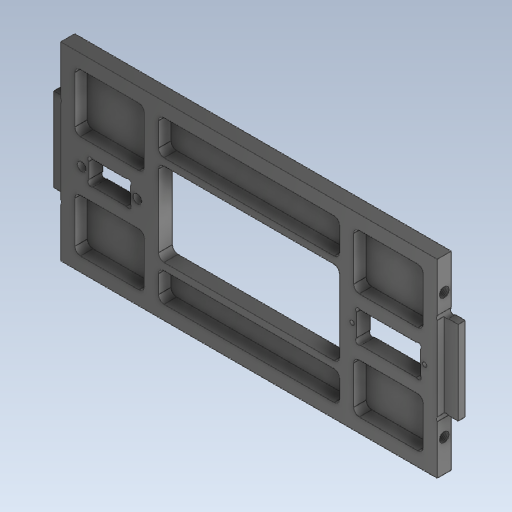
# Autodesk Inventor part: Cockpit_back_frame
Saved by Autodesk Inventor 2020 (Build 240168000, 168)
## iProperties
Part Number: Cockpit_back_frame
Material: アセタール樹脂、黒
Document SubType Name: Modeling
Designer: Masato Kubotera
Density: 1.425 g/cm^3
Appearance: 滑らか - 黒
Description: POM T5
Mass: 27.6157 g
Surface Area: 210.6 cm^2
Volume: 19.3794 cm^3
Author: Masato Kubotera
Autodesk Inventor part; units mm, degrees
ref_plane "XZ Plane" through (0, 0, 0) normal (0, 1, 0) x (-1, 0, 0)
ref_plane "XY Plane" through (0, 0, 0) normal (0, 0, 1) x (1, 0, 0)
derived "Cockpit_side_frame.ipt"
sketch "スケッチ2" plane through (0, 0, 0) normal (0, 1, 0) x (-1, 0, 0)
  line L0 (-23.5, -22.5) -> (-28.5, -27.5)
  line L1 (-28.5, -27.5) -> (-28.5, -91)
  line L2 (-28.5, -91) -> (-23.5, -96)
  line L3 (-23.5, -96) -> (35.75, -96)
  line L4 (37.75, -98) -> (37.75, -131)
  line L5 (37.75, -131) -> (42.75, -136)
  line L6 (42.75, -136) -> (83.5, -136)
  line L7 (88.5, -131) -> (88.5, -20)
  line L8 (88.5, -20) -> (86, -17.5)
  line L9 (86, -17.5) -> (80.25, -17.5)
  line L10 (80.25, -17.5) -> (80.25, -22.5)
  line L11 (80.25, -22.5) -> (73.9849, -22.5)
  line L12 (72.5, -21.0151) -> (72.5, -17.5)
  line L13 (72.5, -17.5) -> (64.5, -17.5)
  line L14 (64.5, -17.5) -> (64.5, -21.0151)
  line L15 (63.0151, -22.5) -> (-23.5, -22.5)
  line L16 (-25.25, -25) -> (-20.25, -25) construction
  line L17 (-20.25, -25) -> (-20.25, -93.5) construction
  line L18 (-20.25, -93.5) -> (-25.25, -93.5) construction
  line L19 (-25.25, -93.5) -> (-25.25, -25) construction
  line L20 (-26, -25) -> (-25.25, -25) construction
  line L21 (-25.25, -93.5) -> (-26, -93.5) construction
  line L22 (-26, -93.5) -> (-26, -25) construction
  line L23 (-20.25, -93.5) -> (80.25, -93.5) construction
  line L24 (-20.25, -88.5) -> (80.25, -88.5) construction
  line L25 (80.25, -22.5) -> (80.25, -90.5) construction
  line L26 (80.25, -90.5) -> (85.25, -90.5) construction
  line L27 (85.25, -90.5) -> (85.25, -22.5) construction
  line L28 (80.25, -88.5) -> (80.25, -93.5) construction
  line L29 (80.25, -91) -> (85.25, -91) construction
  line L30 (85.25, -91) -> (85.25, -133.5) construction
  line L31 (80.25, -91) -> (80.25, -133.5) construction
  line L32 (80.25, -133.5) -> (85.25, -133.5) construction
  line L33 (40.25, -133.5) -> (40.25, -128.5) construction
  line L34 (40.25, -128.5) -> (40.25, -93.5) construction
  line L35 (45.25, -93.5) -> (45.25, -128.5) construction
  line L36 (40.25, -128.5) -> (45.25, -128.5) construction
  line L37 (42.75, -128.5) -> (42.75, -93.5) construction
  line L38 (40.25, -128.5) -> (79.1145, -128.5) construction
  line L39 (79.1145, -128.5) -> (79.1145, -133.5) construction
  line L40 (79.1145, -133.5) -> (40.25, -133.5) construction
  line L41 (40.25, -131) -> (79.1145, -131) construction
  line L42 (82.75, -91) -> (82.75, -133.5) construction
  circle A0 centre (82.75, -131) radius 2
  arc A1 (80.25, -128.5) -> (85.25, -128.5) centre (82.75, -131) ccw construction
  line L43 (80.25, -91) -> (-20.25, -91) construction
  line L44 (42.75, -111) -> (45.25, -111) construction
  line L45 (59.6822, -128.5) -> (59.6822, -131) construction
  line L46 (42.7, -115.5651) -> (42.7, -106.4349)
  line L47 (45.3, -107.05) -> (45.3, -114.95)
  line L48 (45.3, -117.05) -> (42.7, -104.95) construction
  line L49 (42.7, -117.05) -> (45.3, -104.95) construction
  line L50 (55.7322, -128.45) -> (63.6322, -128.45)
  line L51 (64.2473, -131.05) -> (55.1172, -131.05)
  line L52 (53.6322, -128.45) -> (65.7322, -131.05) construction
  line L53 (65.7322, -128.45) -> (53.6322, -131.05) construction
  line L54 (42.75, -105) -> (45.25, -105) construction
  line L55 (42.75, -117) -> (45.25, -117) construction
  arc A2 (44.1849, -104.95) -> (42.7, -106.4349) centre (43.4425, -105.6925) ccw
  arc A3 (45.3, -107.05) -> (45.3, -104.95) centre (45.3, -106) ccw
  arc A4 (42.7, -115.5651) -> (44.1849, -117.05) centre (43.4425, -116.3075) ccw
  arc A5 (45.3, -117.05) -> (45.3, -114.95) centre (45.3, -116) ccw
  line L56 (53.6822, -131) -> (53.6822, -128.5) construction
  line L57 (65.6822, -128.5) -> (65.6822, -131) construction
  arc A6 (53.6322, -129.5651) -> (55.1172, -131.05) centre (54.3747, -130.3075) ccw
  arc A7 (55.7322, -128.45) -> (53.6322, -128.45) centre (54.6822, -128.45) ccw
  arc A8 (64.2473, -131.05) -> (65.7322, -129.5651) centre (64.9898, -130.3075) ccw
  arc A9 (65.7322, -128.45) -> (63.6322, -128.45) centre (64.6822, -128.45) ccw
  line L58 (53.6322, -129.5651) -> (53.6322, -128.45)
  line L59 (65.7322, -128.45) -> (65.7322, -129.5651)
  line L60 (44.1849, -104.95) -> (45.3, -104.95)
  line L61 (45.3, -117.05) -> (44.1849, -117.05)
  circle A10 centre (47.6822, -131) radius 1.6
  line L62 (85.25, -22.5) -> (85.25, -17.5) construction
  line L63 (86, -17.5) -> (86, -90.5) construction
  line L64 (86, -90.5) -> (85.25, -90.5) construction
  line L65 (-18.5, -82.5) -> (-18.5, -61)
  arc A11 (-18.5, -82.5) -> (-16.5, -84.5) centre (-16.5, -82.5) ccw
  line L66 (45.5, -84.5) -> (-16.5, -84.5)
  arc A12 (45.5, -84.5) -> (47.5, -82.5) centre (45.5, -82.5) ccw
  line L67 (47.5, -61) -> (47.5, -82.5)
  arc A13 (47.5, -61) -> (45.5, -59) centre (45.5, -61) ccw
  line L68 (-16.5, -59) -> (45.5, -59)
  arc A14 (-16.5, -59) -> (-18.5, -61) centre (-16.5, -61) ccw
  line L69 (30, -88.5) -> (30, -91) construction
  line L70 (82.75, -22.5) -> (82.75, -90.5) construction
  circle A15 centre (82.75, -34) radius 1.6
  circle A16 centre (82.75, -34) radius 3
  circle A17 centre (82.75, -79) radius 3
  circle A18 centre (82.75, -79) radius 1.6
  line L71 (85.25, -22.5) -> (80.25, -22.5) construction
  arc A19 (85.25, -91) -> (80.25, -91) centre (82.75, -131) ccw construction
  circle A20 centre (47.6822, -131) radius 3
  circle A21 centre (42.75, -99) radius 1.6
  circle A22 centre (42.75, -99) radius 3
  line L72 (5, -88.5) -> (5, -91) construction
  line L73 (55, -88.5) -> (55, -91) construction
  line L74 (53.5651, -91.05) -> (6.4349, -91.05)
  line L75 (4.95, -89.5651) -> (4.95, -88.45)
  line L76 (7.05, -88.45) -> (52.95, -88.45)
  line L77 (55.05, -88.45) -> (55.05, -89.5651)
  line L78 (55.05, -91.05) -> (4.95, -88.45) construction
  line L79 (4.95, -91.05) -> (55.05, -88.45) construction
  arc A23 (7.05, -88.45) -> (4.95, -88.45) centre (6, -88.45) ccw
  arc A24 (4.95, -89.5651) -> (6.4349, -91.05) centre (5.6925, -90.3075) ccw
  arc A25 (53.5651, -91.05) -> (55.05, -89.5651) centre (54.3075, -90.3075) ccw
  arc A26 (55.05, -88.45) -> (52.95, -88.45) centre (54, -88.45) ccw
  line L80 (-20.25, -41) -> (80.25, -41) construction
  line L81 (80.25, -36) -> (-20.25, -36) construction
  line L82 (-20.25, -36) -> (-20.25, -41) construction
  line L83 (-20.25, -38.5) -> (80.25, -38.5) construction
  line L84 (30, -41) -> (30, -36) construction
  line L85 (53.5651, -35.95) -> (6.4349, -35.95)
  line L86 (6.4349, -41.05) -> (53.5651, -41.05)
  line L87 (55.05, -35.95) -> (4.95, -41.05) construction
  line L88 (4.95, -35.95) -> (55.5723, -41.1032) construction
  arc A27 (6.4349, -35.95) -> (4.95, -37.4349) centre (5.6925, -36.6925) ccw
  arc A28 (4.95, -39.5651) -> (6.4349, -41.05) centre (5.6925, -40.3075) ccw
  arc A29 (55.05, -37.4349) -> (53.5651, -35.95) centre (54.3075, -36.6925) ccw
  arc A30 (53.5651, -41.05) -> (55.05, -39.5651) centre (54.3075, -40.3075) ccw
  line L89 (5, -41) -> (5, -36) construction
  line L90 (55, -36) -> (55, -41) construction
  line L91 (4.95, -37.4349) -> (4.95, -39.5651)
  line L92 (55.05, -39.5651) -> (55.05, -37.4349)
  circle A31 centre (-2.5, -38.5) radius 1.6
  circle A32 centre (-2.5, -38.5) radius 3
  circle A33 centre (62.5, -38.5) radius 1.6
  circle A34 centre (62.5, -38.5) radius 3
  line L93 (-25.25, -44.25) -> (-22.75, -44.25) construction
  line L94 (-25.25, -49.25) -> (-26, -49.25) construction
  line L95 (-25.25, -74.25) -> (-22.75, -74.25) construction
  line L96 (-25.25, -69.25) -> (-26, -69.25) construction
  line L97 (-26, -59.25) -> (-25.25, -59.25) construction
  line L98 (-25.25, -59.25) -> (-22.75, -59.25) construction
  line L99 (-22.75, -25) -> (-22.75, -93.5) construction
  arc A35 (63.0151, -22.5) -> (64.5, -21.0151) centre (63.7575, -21.7575) ccw
  arc A36 (72.5, -21.0151) -> (73.9849, -22.5) centre (73.2425, -21.7575) ccw
  line L100 (56.75, -22.5) -> (56.75, -32.5) construction
  line L101 (56.75, -32.5) -> (80.25, -32.5) construction
  line L102 (80.25, -32.5) -> (80.25, -22.5) construction
  line L103 (68.5, -17.5) -> (68.5, -32.5) construction
  line L104 (60.5, -22.5) -> (60.5, -17.5) construction
  line L105 (76.5, -22.5) -> (76.5, -17.5) construction
  line L106 (-22.7, -46.3) -> (-22.7, -72.2)
  line L107 (-25.3, -72.8151) -> (-25.3, -69.564)
  line L108 (-25.3, -44.2) -> (-22.7, -74.3) construction
  line L109 (-22.7, -44.2) -> (-25.3, -74.3) construction
  arc A37 (-22.7, -46.3) -> (-22.7, -44.2) centre (-22.7, -45.25) ccw
  arc A38 (-23.8151, -44.2) -> (-25.3, -45.6849) centre (-24.5575, -44.9425) ccw
  line L110 (-23.8151, -44.2) -> (-22.7, -44.2)
  arc A39 (-25.3, -72.8151) -> (-23.8151, -74.3) centre (-24.5575, -73.5575) ccw
  arc A40 (-22.7, -74.3) -> (-22.7, -72.2) centre (-22.7, -73.25) ccw
  line L111 (-22.7, -74.3) -> (-23.8151, -74.3)
  line L112 (-26.3, -49.9848) -> (-26.3, -68.5152)
  arc A41 (-26.3, -68.5152) -> (-25.3, -69.564) centre (-25.25, -68.5152) ccw
  arc A42 (-25.3, -48.936) -> (-26.3, -49.9848) centre (-25.25, -49.9848) ccw
  line L113 (-25.3, -48.936) -> (-25.3, -45.6849)
  circle A43 centre (-22.75, -36.75) radius 1.6
  circle A44 centre (-22.75, -36.75) radius 3
  circle A45 centre (-22.75, -81.75) radius 1.6
  circle A46 centre (-22.75, -81.75) radius 3
  line L114 (64.5, -22.5) -> (72.5, -22.5)
  line L115 (85.25, -17.5) -> (52.5, -17.5) construction
  line L116 (52.5, -17.5) -> (52.5, -22.5) construction
  circle A47 centre (82.75, -93.5) radius 1.475
  circle A48 centre (82.75, -98.5) radius 1.475
  circle A49 centre (82.75, -103.5) radius 1.475
  line L117 (49.75, -93.5) -> (78.25, -93.5)
  line L118 (80.25, -95.5) -> (80.25, -124)
  line L119 (78.25, -126) -> (49.75, -126)
  line L120 (47.75, -124) -> (47.75, -95.5)
  arc A50 (49.75, -93.5) -> (47.75, -95.5) centre (49.75, -95.5) ccw
  arc A51 (47.75, -124) -> (49.75, -126) centre (49.75, -124) ccw
  arc A52 (78.25, -126) -> (80.25, -124) centre (78.25, -124) ccw
  arc A53 (80.25, -95.5) -> (78.25, -93.5) centre (78.25, -95.5) ccw
  arc A54 (37.75, -98) -> (35.75, -96) centre (35.75, -98) ccw
  circle A55 centre (-13.5, -55) radius 1.75
  circle A56 centre (-13.5, -55) radius 2
  line L121 (74.85, -78.65) -> (65.65, -78.65) construction
  line L122 (65.65, -78.65) -> (65.65, -64.85) construction
  line L123 (65.65, -64.85) -> (74.85, -64.85) construction
  line L124 (74.85, -64.85) -> (74.85, -78.65) construction
  line L125 (74.85, -78.65) -> (65.65, -64.85) construction
  line L126 (65.65, -78.65) -> (74.85, -64.85) construction
  line L127 (64.95, -64.2) -> (75.55, -64.2) construction
  line L128 (75.55, -64.2) -> (75.55, -79.3) construction
  line L129 (75.55, -79.3) -> (64.95, -79.3) construction
  line L130 (64.95, -79.3) -> (64.95, -64.2) construction
  line L131 (64.95, -64.2) -> (75.55, -79.3) construction
  line L132 (75.55, -64.2) -> (64.95, -79.3) construction
  line L133 (66.3849, -64.15) -> (74.1151, -64.15)
  line L134 (75.6, -65.6349) -> (75.6, -77.8651)
  line L135 (75.6, -79.35) -> (64.9, -64.15) construction
  line L136 (64.9, -79.35) -> (75.6, -64.15) construction
  line L137 (74.9, -78.7) -> (65.6, -64.8) construction
  line L138 (65.6, -78.7) -> (74.9, -64.8) construction
  arc A57 (66.3849, -64.15) -> (64.9, -65.6349) centre (65.6425, -64.8925) ccw
  arc A58 (67.0849, -64.8) -> (65.6, -66.2849) centre (66.3425, -65.5425) ccw
  line L139 (64.9, -71.75) -> (75.6, -71.75) construction
  line L140 (70.25, -64.15) -> (70.25, -78.7063) construction
  arc A59 (75.6, -65.6349) -> (74.1151, -64.15) centre (74.8575, -64.8925) ccw
  arc A60 (74.9, -66.2849) -> (73.4151, -64.8) centre (74.1575, -65.5425) ccw
  arc A61 (65.6, -77.2151) -> (67.0849, -78.7) centre (66.3425, -77.9575) ccw
  arc A62 (64.9, -77.8651) -> (66.3849, -79.35) centre (65.6425, -78.6075) ccw
  arc A63 (73.4151, -78.7) -> (74.9, -77.2151) centre (74.1575, -77.9575) ccw
  arc A64 (74.1151, -79.35) -> (75.6, -77.8651) centre (74.8575, -78.6075) ccw
  line L141 (67.0849, -64.8) -> (73.4151, -64.8)
  line L142 (74.9, -66.2849) -> (74.9, -77.2151)
  line L143 (64.9, -77.8651) -> (64.9, -65.6349)
  line L144 (65.6, -77.2151) -> (65.6, -66.2849)
  line L145 (73.4151, -78.7) -> (67.0849, -78.7)
  line L146 (74.1151, -79.35) -> (66.3849, -79.35)
  line L147 (-18.5, -71.75) -> (47.5, -71.75) construction
  line L148 (82.75, -56.5) -> (85.25, -56.5) construction
  line L149 (86, -54) -> (85.25, -54) construction
  line L150 (82.7, -69.45) -> (82.7, -43.55)
  line L151 (85.3057, -71.616) -> (82.7, -41.45) construction
  line L152 (82.7, -71.55) -> (85.3, -41.45) construction
  arc A65 (82.7, -41.45) -> (82.7, -43.55) centre (82.7, -42.5) ccw
  arc A66 (85.3, -42.9349) -> (83.8151, -41.45) centre (84.5575, -42.1925) ccw
  arc A67 (82.7, -69.45) -> (82.7, -71.55) centre (82.7, -70.5) ccw
  arc A68 (83.8151, -71.55) -> (85.3, -70.0651) centre (84.5575, -70.8075) ccw
  line L153 (82.75, -41.5) -> (85.25, -41.5) construction
  line L154 (82.75, -71.5) -> (85.25, -71.5) construction
  arc A69 (86.25, -47.1801) -> (85.3, -46.1348) centre (85.2, -47.1801) ccw
  line L155 (86.25, -47.1801) -> (86.25, -65.8199)
  line L156 (85.25, -46.5) -> (86, -46.5) construction
  line L157 (85.25, -66.5) -> (86, -66.5) construction
  arc A70 (85.3, -66.8652) -> (86.25, -65.8199) centre (85.2, -65.8199) ccw
  line L158 (85.3, -42.9349) -> (85.3, -46.1348)
  line L159 (85.3, -66.8652) -> (85.3, -70.0651)
  line L160 (83.8151, -71.55) -> (82.7, -71.55)
  line L161 (82.7, -41.45) -> (83.8151, -41.45)
  line L162 (83.5, -136) -> (88.5, -131)
  point P0 (0, 0)
  point P1 (-25.7227, -96)
  point P2 (-23.5, -22.5)
  point P3 (44, -111)
  point P4 (59.6822, -129.75)
  point P5 (30, -89.75)
  point P6 (30, -38.5)
  point P7 (4.95, -41.05)
  point P8 (52.5, -22)
  point P9 (-24, -59.25)
  point P10 (70.25, -71.75)
  point P11 (70.25, -71.75)
  point P12 (84, -56.5)
  dimension "d2" = 85.25
  dimension "d10" = 2.5
  dimension "d11" = 5
  measures "d2" distance from line of L27 point (0, 0)
  measures "d10" distance of L154.start L154.end
  measures "d11" distance of L25.end L26.end
ref_plane "作業平面1" through (-85.25, 0, 0) normal (1, 0, 0) x (0, 1, 0)
sketch "スケッチ3" plane through (-85.25, 0, 0) normal (1, 0, 0) x (0, 1, 0)
  line L0 (-135, -22.5) -> (0, -22.5)
  line L1 (0, -22.5) -> (0, -40.0151)
  line L2 (0, -90.5) -> (-135, -90.5)
  line L3 (-135, -56.5) -> (0, -56.5) construction
  line L4 (-67.5, -22.5) -> (-67.5, -90.5) construction
  line L5 (1.4849, -41.5) -> (5, -41.5)
  line L6 (5, -41.5) -> (5, -71.5)
  line L7 (5, -71.5) -> (1.4849, -71.5)
  arc A0 (0, -40.0151) -> (1.4849, -41.5) centre (0.7425, -40.7575) ccw
  arc A1 (1.4849, -71.5) -> (0, -72.9849) centre (0.7425, -72.2425) ccw
  line L8 (0, -41.5) -> (0, -71.5)
  line L9 (0, -72.9849) -> (0, -90.5)
  line L10 (-135, -22.5) -> (-135, -40.0151)
  line L11 (-136.4849, -41.5) -> (-140, -41.5)
  line L12 (-140, -41.5) -> (-140, -71.5)
  line L13 (-140, -71.5) -> (-136.4849, -71.5)
  arc A2 (-136.4849, -41.5) -> (-135, -40.0151) centre (-135.7425, -40.7575) ccw
  arc A3 (-135, -72.9849) -> (-136.4849, -71.5) centre (-135.7425, -72.2425) ccw
  line L14 (-135, -41.5) -> (-135, -71.5)
  line L15 (-135, -72.9849) -> (-135, -90.5)
  line L16 (-98, -42.5) -> (-37, -42.5)
  line L17 (-35, -44.5) -> (-35, -70.5)
  line L18 (-37, -72.5) -> (-98, -72.5)
  line L19 (-100, -70.5) -> (-100, -44.5)
  arc A4 (-98, -42.5) -> (-100, -44.5) centre (-98, -44.5) ccw
  arc A5 (-100, -70.5) -> (-98, -72.5) centre (-98, -70.5) ccw
  arc A6 (-37, -72.5) -> (-35, -70.5) centre (-37, -70.5) ccw
  arc A7 (-35, -44.5) -> (-37, -42.5) centre (-37, -44.5) ccw
  line L20 (-109.75, -53.45) -> (-125.25, -53.45) construction
  line L21 (-125.25, -53.45) -> (-125.25, -61.55) construction
  line L22 (-125.25, -61.55) -> (-109.75, -61.55) construction
  line L23 (-109.75, -61.55) -> (-109.75, -53.45) construction
  line L24 (-109.75, -53.45) -> (-125.25, -61.55) construction
  line L25 (-125.25, -53.45) -> (-109.75, -61.55) construction
  line L26 (-125, -61.8) -> (-110, -61.8)
  line L27 (-110, -61.8) -> (-110, -53.2)
  line L28 (-110, -53.2) -> (-125, -53.2)
  line L29 (-125, -53.2) -> (-125, -61.8)
  line L30 (-125, -61.8) -> (-110, -53.2) construction
  line L31 (-110, -61.8) -> (-125, -53.2) construction
  line L32 (-107.5, -57.5) -> (-127.5, -57.5) construction
  line L33 (-117.5, -53.2) -> (-117.5, -61.8) construction
  circle A8 centre (-107.5, -57.5) radius 1.6
  circle A9 centre (-107.5, -57.5) radius 2.25 construction
  circle A10 centre (-127.5, -57.5) radius 1.6
  line L34 (-28.75, -62.75) -> (-6.25, -62.75) construction
  line L35 (-29, -63) -> (-6, -63)
  line L36 (-28.75, -52.25) -> (-28.75, -62.75) construction
  line L37 (-6.25, -62.75) -> (-6.25, -52.25) construction
  line L38 (-6.25, -52.25) -> (-28.75, -52.25) construction
  line L39 (-28.75, -52.25) -> (-6.25, -62.75) construction
  line L40 (-28.75, -62.75) -> (-6.25, -52.25) construction
  line L41 (-17.5, -52.25) -> (-17.5, -62.75) construction
  line L42 (-29, -52) -> (-29, -63)
  line L43 (-6, -63) -> (-6, -52)
  line L44 (-6, -52) -> (-29, -52)
  line L45 (-29, -52) -> (-6, -63) construction
  line L46 (-29, -63) -> (-6, -52) construction
  circle A11 centre (-4.5, -57.5) radius 0.8
  arc A12 (-6, -53.4849) -> (-7.4849, -52) centre (-6.7425, -52.7425) ccw
  arc A13 (-7.4849, -63) -> (-6, -61.5151) centre (-6.7425, -62.2575) ccw
  line L47 (-30.5, -57.5) -> (-4.5, -57.5) construction
  arc A14 (-29, -61.5151) -> (-27.5151, -63) centre (-28.2575, -62.2575) ccw
  circle A15 centre (-30.5, -57.5) radius 0.8
  arc A16 (-27.5151, -52) -> (-29, -53.4849) centre (-28.2575, -52.7425) ccw
  arc A17 (-110, -54.6849) -> (-111.4849, -53.2) centre (-110.7425, -53.9425) ccw
  arc A18 (-123.5151, -53.2) -> (-125, -54.6849) centre (-124.2575, -53.9425) ccw
  arc A19 (-125, -60.3151) -> (-123.5151, -61.8) centre (-124.2575, -61.0575) ccw
  arc A20 (-111.4849, -61.8) -> (-110, -60.3151) centre (-110.7425, -61.0575) ccw
  line L48 (-130, -29.5) -> (-130, -46.45)
  line L49 (-128, -48.45) -> (-107, -48.45)
  line L50 (-128, -27.5) -> (-107, -27.5)
  line L51 (-105, -29.5) -> (-105, -46.45)
  line L52 (-28, -27.5) -> (-7, -27.5)
  line L53 (-5, -29.5) -> (-5, -45.25)
  line L54 (-7, -47.25) -> (-28, -47.25)
  line L55 (-30, -45.25) -> (-30, -29.5)
  line L56 (-98, -27.5) -> (-37, -27.5)
  line L57 (-35, -29.5) -> (-35, -38)
  line L58 (-37, -40) -> (-98, -40)
  line L59 (-100, -38) -> (-100, -29.5)
  line L60 (-128, -66.55) -> (-107, -66.55)
  line L61 (-7, -67.75) -> (-28, -67.75)
  line L62 (-37, -75) -> (-98, -75)
  line L63 (-128, -85.5) -> (-107, -85.5)
  line L64 (-28, -85.5) -> (-7, -85.5)
  line L65 (-98, -85.5) -> (-37, -85.5)
  line L66 (-130, -68.55) -> (-130, -83.5)
  line L67 (-105, -68.55) -> (-105, -83.5)
  line L68 (-100, -83.5) -> (-100, -77)
  line L69 (-35, -77) -> (-35, -83.5)
  line L70 (-30, -83.5) -> (-30, -69.75)
  line L71 (-5, -69.75) -> (-5, -83.5)
  arc A21 (-128, -27.5) -> (-130, -29.5) centre (-128, -29.5) ccw
  arc A22 (-130, -46.45) -> (-128, -48.45) centre (-128, -46.45) ccw
  arc A23 (-107, -48.45) -> (-105, -46.45) centre (-107, -46.45) ccw
  arc A24 (-105, -29.5) -> (-107, -27.5) centre (-107, -29.5) ccw
  arc A25 (-98, -27.5) -> (-100, -29.5) centre (-98, -29.5) ccw
  arc A26 (-100, -38) -> (-98, -40) centre (-98, -38) ccw
  arc A27 (-37, -40) -> (-35, -38) centre (-37, -38) ccw
  arc A28 (-35, -29.5) -> (-37, -27.5) centre (-37, -29.5) ccw
  arc A29 (-28, -27.5) -> (-30, -29.5) centre (-28, -29.5) ccw
  arc A30 (-5, -29.5) -> (-7, -27.5) centre (-7, -29.5) ccw
  arc A31 (-7, -47.25) -> (-5, -45.25) centre (-7, -45.25) ccw
  arc A32 (-30, -45.25) -> (-28, -47.25) centre (-28, -45.25) ccw
  arc A33 (-28, -67.75) -> (-30, -69.75) centre (-28, -69.75) ccw
  arc A34 (-30, -83.5) -> (-28, -85.5) centre (-28, -83.5) ccw
  arc A35 (-7, -85.5) -> (-5, -83.5) centre (-7, -83.5) ccw
  arc A36 (-5, -69.75) -> (-7, -67.75) centre (-7, -69.75) ccw
  arc A37 (-37, -85.5) -> (-35, -83.5) centre (-37, -83.5) ccw
  arc A38 (-35, -77) -> (-37, -75) centre (-37, -77) ccw
  arc A39 (-100, -83.5) -> (-98, -85.5) centre (-98, -83.5) ccw
  arc A40 (-98, -75) -> (-100, -77) centre (-98, -77) ccw
  arc A41 (-107, -85.5) -> (-105, -83.5) centre (-107, -83.5) ccw
  arc A42 (-105, -68.55) -> (-107, -66.55) centre (-107, -68.55) ccw
  arc A43 (-128, -66.55) -> (-130, -68.55) centre (-128, -68.55) ccw
  arc A44 (-130, -83.5) -> (-128, -85.5) centre (-128, -83.5) ccw
  point P0 (0, 0)
  point P1 (-135, -71.5)
  point P2 (0, -90.5)
  point P3 (0, -71.5)
  point P4 (0, -41.5)
  point P5 (-67.5, -42.5)
  point P6 (-117.5, -57.5)
  point P7 (-117.5, -57.5)
  point P8 (-17.5, -57.5)
  point P9 (-17.5, -57.5)
  point P10 (-123.5151, -53.2)
  point P11 (-110, -60.3151)
  point P12 (-111.4849, -61.8)
  point P13 (-123.5151, -61.8)
  point P14 (-125, -60.3151)
  point P15 (-27.5151, -63)
  point P16 (-7.4849, -52)
  point P17 (-6, -53.4849)
  point P18 (-6, -61.5151)
  point P19 (-7.4849, -63)
  point P20 (-100, -57.5)
  point P21 (-130, -27.5)
  point P22 (-130, -48.45)
  point P23 (-105, -27.5)
  point P24 (-105, -48.45)
  point P25 (-30, -27.5)
  point P26 (-5, -47.25)
  point P27 (-5, -27.5)
  point P28 (-30, -47.25)
  point P29 (-100, -27.5)
  point P30 (-35, -40)
  point P31 (-35, -27.5)
  point P32 (-100, -40)
  point P33 (-130, -66.55)
  point P34 (-105, -66.55)
  point P35 (-5, -67.75)
  point P36 (-30, -67.75)
  point P37 (-35, -75)
  point P38 (-100, -75)
  point P39 (-130, -85.5)
  point P40 (-105, -85.5)
  point P41 (-30, -85.5)
  point P42 (-5, -85.5)
  point P43 (-100, -85.5)
  point P44 (-35, -85.5)
  dimension "d3" = 1.05
  dimension "d4" = 135
  dimension "d5" = 5
  dimension "d20" = 2
  dimension "d21" = 30
  dimension "d22" = 65
  dimension "d23" = 20
  dimension "d25" = 15.5
  dimension "d26" = 8.1
  dimension "d27" = 0.25
  dimension "d28" = 0.25
  dimension "d29" = 20
  dimension "d30" = 3.2
  dimension "d31" = 4.5
  dimension "d33" = 10.5
  dimension "d34" = 22.5
  dimension "d35" = 26
  dimension "d36" = 1.6
  dimension "d37" = 1.05
  dimension "d38" = 23
  dimension "d39" = 11
  dimension "d41" = 1.05
  dimension "d46" = 17.5
  dimension "d47" = 35
  dimension "d48" = 17.5
  dimension "d49" = 5
  dimension "d50" = 5
  dimension "d51" = 5
  dimension "d52" = 5
  dimension "d53" = 5
  dimension "d54" = 2.5
  dimension "d55" = 2
  constraints: 142 end point, 85 point on circle, 63 point on line, 57 tangent, 45 centre point, 45 symmetric about line, 26 equal radius, 23 parallel, 22 midpoint, 17 perpendicular, 7 horizontal, 5 coincident, 4 collinear, 1 vertical, 17 other
  measures "d3" radius of A0
  measures "d4" distance of L0.start L0.end
  measures "d5" distance of L8.start L5.end
  measures "d20" radius of A4
  measures "d21" distance between parallel lines of L18 L16
  measures "d22" distance between parallel lines of L17 L19
  measures "d23" distance between parallel lines of L16 L0
  measures "d25" distance of L23.start L21.end
  measures "d26" distance of L21.end L21.start
  measures "d27" horizontal distance of L28.start L20.start
  measures "d28" horizontal distance of L28.start L20.start
  measures "d29" distance of L32.start L32.end
  measures "d30" diameter of A8
  measures "d31" diameter of A9
  measures "d33" distance of L38.start L34.end
  measures "d34" distance of L34.end L34.start
  measures "d35" distance of L47.start L47.end
  measures "d36" diameter of A15
  measures "d37" radius of A16
  measures "d38" distance of L44.start L44.end
  measures "d39" distance of L44.end L35.start
  measures "d41" radius of A17
  measures "d46" distance between parallel lines of L19 L33
  measures "d47" distance between parallel lines of L14 L19
  measures "d48" distance between parallel lines of L17 L41
  measures "d49" distance between parallel lines of L0 L56
  measures "d50" distance between parallel lines of L10 L48
  measures "d51" distance between parallel lines of L51 L59
  measures "d52" distance between parallel lines of L49 L20
  measures "d53" distance between parallel lines of L38 L54
  measures "d54" distance between parallel lines of L16 L58
  measures "d55" radius of A21
extrude "押し出し1" add sketch "スケッチ3" along normal blind 5 contours L0 L1 A0 L8 A1 L9 L2 L15 A3 L14 A2 L10
extrude "押し出し2" add sketch "スケッチ3" along normal blind 2.5 contours L14 A3 L13 L12 L11 A2 | A0 L5 L6 L7 A1 L8
hole "穴1" at (28.5, 0, -27.5) at (25.7227, 0, -96) at (23.5, 0, -22.5) at (-52.5, 0, -22) at (13.5, 0, -55) at (-82.75, 0, -79) at (-82.75, 0, -34) direction (0, -1, 0) diameter 3.4587 depth 4 thread size "M4x0.5" class "6H" standard "ISO Metric profile"
ref_plane "作業平面2" through (-85.25, -67.5, -22.5) normal (0, 1, 0) x (1, 0, 0)
mirror "ミラー1" about plane through (-85.25, -67.5, -22.5) normal (0, 1, 0) of "穴1"
extrude "押し出し3" add sketch "スケッチ3" along normal blind 0.5 contours A21 L50 A24 L51 A23 L49 A22 L48 | L52 A30 L53 A31 L54 A32 L55 A29 | L56 A28 L57 A27 L58 A26 L59 A25 | L60 A42 L67 A41 L63 A44 L66 A43 | A36 L71 A35 L64 A34 L70 A33 L61 | A38 L69 A37 L65 A39 L68 A40 L62
equation "\"d28\" = d27"
equation "\"d41\" = d42"
equation "\"d6\" = d11"
equation "\"d8\" = d10"
equation "\"d1\" = -d2"
equation "\"d42\" = 1.05"
